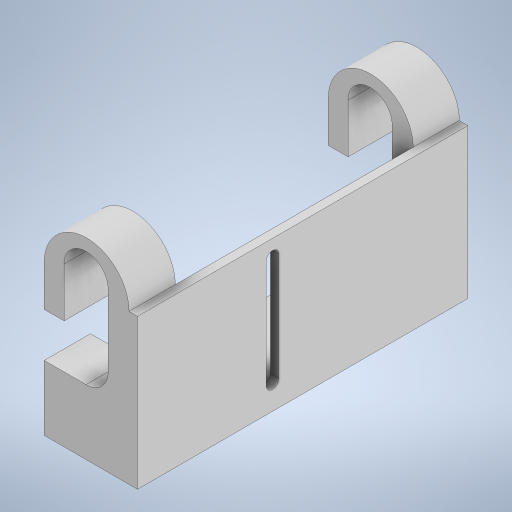
# Autodesk Inventor part: 6 Backet Adjustment 3.0
Saved by Autodesk Inventor 2024 (Build 280153000, 153)
## iProperties
Created: 2023-10-21
Part Number: 6 Backet Adjustment 3.0
Material: Generic
Document SubType Name: Modeling
Designer: olson
Density: 1 g/cm^3
Appearance: Default
Author: olson
Autodesk Inventor part; units mm, degrees
ref_plane "YZ Plane" through (0, 0, 0) normal (1, 0, 0) x (0, 1, 0)
ref_plane "XZ Plane" through (0, 0, 0) normal (0, 1, 0) x (-1, 0, 0)
ref_plane "XY Plane" through (0, 0, 0) normal (0, 0, 1) x (1, 0, 0)
sketch "Sketch1" plane through (0, 0, 0) normal (0, 1, 0) x (-1, 0, 0)
  line L0 (10, 67.88) -> (-10, 67.88)
  line L1 (-10, 67.88) -> (-10, -10)
  line L2 (-10, -10) -> (10, -10)
  line L3 (10, -10) -> (10, 67.88)
  point P0 (0, 0)
  dimension "d0" = 20
  dimension "d1" = 77.88
  constraints: 8 end point, 2 parallel, 1 horizontal, 1 perpendicular
  measures "d0" distance of L2.end L1.end
  measures "d1" distance of L1.end L0.end
extrude "Extrusion1" add sketch "Sketch1" along normal blind 2
sketch "Sketch2" plane through (0, 2, 0) normal (0, 1, 0) x (1, 0, 0)
  line L0 (-10, -67.88) -> (10, -67.88) projected
  line L1 (0, -67.88) -> (-6.35, -67.88)
  line L2 (-6.35, -56.98) -> (6.35, -56.98)
  line L3 (6.35, -67.88) -> (0, -67.88)
  line L4 (10, 10) -> (-10, 10) projected
  line L5 (-6.35, -0.9) -> (6.35, -0.9)
  line L6 (-6.35, 10) -> (6.35, 10)
  line L7 (-6.35, -67.88) -> (-10, -67.88)
  line L8 (-10, 10) -> (-10, -67.88) projected
  line L9 (-10, -56.98) -> (-6.35, -56.98)
  line L10 (6.35, -67.88) -> (10, -67.88)
  line L11 (10, -67.88) -> (10, 10) projected
  line L12 (10, -56.98) -> (6.35, -56.98)
  line L13 (6.35, -0.9) -> (10, -0.9)
  line L14 (10, 10) -> (6.35, 10)
  line L15 (10, -0.9) -> (10, 10)
  line L16 (10, -67.88) -> (10, -56.98)
  line L17 (-10, -67.88) -> (-10, -56.98)
  line L18 (-6.35, -0.9) -> (-10, -0.9)
  line L19 (-10, -0.9) -> (-10, 10)
  line L20 (-10, 10) -> (-6.35, 10)
  point P0 (0, 0)
  dimension "d4" = 6.35
  dimension "d5" = 10.9
  dimension "d6" = 12.7
  dimension "d7" = 10.9
  constraints: 34 end point, 9 point on line, 7 perpendicular, 4 collinear, 1 horizontal, 1 midpoint, 1 parallel, 1 vertical
  measures "d4" distance of L1.start L1.end
  measures "d5" distance of L1.end L2.start
  measures "d6" distance of L2.start L2.end
  measures "d7" distance of L6.start L5.start
extrude "Extrusion2" add sketch "Sketch2" along normal blind 43.3354 contours L8 L9 L2 L12 L11 L0 | L8 L4 L11 L13 L5 L18
sketch "Sketch9" plane through (-10, 0, 67.88) normal (0, 0, 1) x (1, 0, 0)
  arc A0 (15.084, 37.3223) -> (4.684, 37.3223) centre (9.884, 37.3223) ccw
  line L0 (15.084, 30.9243) -> (15.084, 37.3223)
  line L1 (4.684, 36.1247) -> (4.684, 37.3223)
  arc A1 (15.084, 37.3223) -> (4.684, 37.3223) centre (9.884, 37.3223) ccw
  line L2 (4.684, 37.3223) -> (4.684, 30.9247)
  line L3 (9.8815, 15.3222) -> (-0.0013, 15.3222)
  line L4 (-0.0013, 25.726) -> (-0.0013, 15.3222)
  line L5 (4.684, 30.9247) -> (4.684, 25.726)
  line L6 (15.084, 30.9243) -> (15.0845, 20.5254)
  arc A2 (15.084, 30.9243) -> (15.084, 30.9251) centre (9.884, 30.9244) ccw
  line L7 (4.684, 25.726) -> (-0.0013, 25.726)
  arc A3 (9.8815, 15.3222) -> (15.0845, 20.5254) centre (9.8815, 20.5252) ccw
  line L8 (0, 0) -> (20, 0) projected
  line L9 (0, 45.3354) -> (20, 45.3354) projected
  point P0 (10, 0)
  point P1 (2.3413, 25.726)
  point P2 (15.084, 30.9247)
  point P3 (9.884, 42.5223)
  point P4 (-0.0013, 20.5241)
  point P5 (10, 45.3354)
  dimension "d76" = 15.3222
  dimension "d77" = 10.4039
  dimension "d78" = 10.4
  dimension "d79" = 27.2001
  dimension "d80" = 15.0858
  dimension "d81" = 8.0131
  constraints: 16 end point, 10 point on circle, 4 centre point, 3 midpoint, 3 tangent, 2 horizontal, 2 perpendicular, 2 point on line, 1 coincident, 1 vertical
  measures "d76" distance between parallel lines of L8 L3
  measures "d77" distance from line of L3 point (2.341, 25.726)
  measures "d78" distance of point (15.084, 30.925) L2.end
  measures "d79" distance from line of L3 point (9.884, 42.522)
  measures "d80" distance from line of L6 point (-0.001, 20.524)
  measures "d81" vertical distance of point (10, 45.335) A1.centre
fillet "Fillet4" radius 10 4 edges at (10, 45.3354, 62.43) (-10, 45.3354, 62.43) (-10, 45.3354, -4.55) (10, 45.3354, -4.55)
sketch "Sketch10" plane through (0, 2, 0) normal (0, 1, 0) x (1, 0, 0)
  line L0 (10, -67.88) -> (-10, -67.88) projected
  line L1 (-10, 10) -> (10, 10) projected
  line L2 (10, -56.98) -> (10, -0.9) projected
  line L3 (-10, -0.9) -> (-10, -56.98) projected
  line L4 (10, -28.94) -> (-10, -28.94)
  circle A0 centre (0, -28.94) radius 2.125
  point P0 (0, 0)
  dimension "d53" = 77.88
  dimension "d54" = 4.25
  constraints: 3 midpoint, 2 end point, 1 centre point
  measures "d53" distance between parallel lines of L0 L1
  measures "d54" diameter of A0
extrude "Extrusion10" cut sketch "Sketch10" against normal blind 2
extrude "Extrusion11" cut sketch "Sketch9" against normal through all
sketch "Sketch11" plane through (10, 0, 67.88) normal (1, 0, 0) x (0, 0, -1)
  line L0 (0, 0) -> (0, 15.3222) projected
  line L1 (77.88, 25.726) -> (77.88, 35.3354) projected
  line L2 (0, 0) -> (77.88, 0)
  line L3 (77.88, 0) -> (77.88, 35.3354)
  line L4 (77.88, 35.3354) -> (0, 35.3354)
  line L5 (0, 35.3354) -> (0, 0)
  point P0 (67.88, 0)
  constraints: 8 end point, 2 parallel, 1 horizontal, 1 perpendicular
extrude "Extrusion12" add sketch "Sketch11" along normal blind 2
sketch "Sketch12" plane through (12, 0, 67.88) normal (1, 0, 0) x (0, 0, -1)
  line L0 (10.9, 35.3354) -> (0, 35.3354) projected
  line L1 (77.88, 25.726) -> (77.88, 35.3354) projected
  line L2 (0, 35.3354) -> (77.88, 35.3354)
  line L3 (77.88, 35.3354) -> (0, 35.3354) projected
  line L4 (38.94, 35.3354) -> (64.34, 35.3354)
  line L5 (38.94, 35.3354) -> (13.54, 35.3354)
  line L6 (77.88, 0) -> (0, 0) projected
  line L7 (13.54, 35.3354) -> (64.34, 35.3354)
  line L8 (64.34, 35.3354) -> (64.34, 0)
  line L9 (64.34, 0) -> (13.54, 0)
  line L10 (13.54, 0) -> (13.54, 35.3354)
  line L11 (13.54, 0) -> (31.84, 0)
  line L12 (31.84, 0) -> (31.84, 6)
  arc A0 (33.34, 31.3354) -> (30.34, 31.3354) centre (31.84, 31.3354) ccw
  arc A1 (30.34, 6) -> (33.34, 6) centre (31.84, 6) ccw
  line L13 (30.34, 31.3354) -> (30.34, 6)
  line L14 (33.34, 31.3354) -> (33.34, 6)
  line L15 (31.84, 31.3354) -> (13.54, 31.3354)
  point P0 (67.88, 0)
  dimension "d65" = 25.4
  dimension "d66" = 25.4
  dimension "d67" = 50.8
  dimension "d68" = 18.3
  dimension "d69" = 6
  dimension "d71" = 3
  dimension "d72" = 3
  dimension "d75" = 18.3
  constraints: 24 end point, 5 point on line, 4 point on circle, 2 centre point, 2 horizontal, 2 parallel, 2 perpendicular, 2 tangent, 1 coincident, 1 midpoint, 1 vertical
  measures "d65" distance of L4.start L4.end
  measures "d66" distance of L4.start L5.end
  measures "d67" distance of L8.end L9.end
  measures "d68" distance of L9.end L11.end
  measures "d69" distance of L11.end L12.end
  measures "d71" diameter of A0
  measures "d72" diameter of A1
  measures "d75" distance of L15.start L15.end
extrude "Extrusion13" cut sketch "Sketch12" against normal blind 2 contours A0 L14 A1 L13
body "Solid1"
